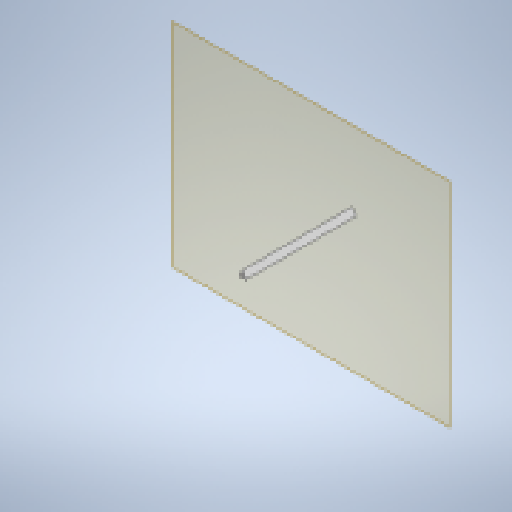
# Autodesk Inventor part: Pieza6
Saved by Autodesk Inventor 2024 (Build 280153000, 153)
## iProperties
Created: 2025-08-12
Part Number: Pieza6
Material: Genérico
Document SubType Name: Modeling
Designer: sergi
Density: 1 g/cm^3
Appearance: Valor por defecto
Author: sergi
Autodesk Inventor part; units mm, degrees
ref_plane "YZ Plane" through (0, 0, 0) normal (1, 0, 0) x (0, 1, 0)
ref_plane "XZ Plane" through (0, 0, 0) normal (0, 1, 0) x (-1, 0, 0)
ref_plane "XY Plane" through (0, 0, 0) normal (0, 0, 1) x (1, 0, 0)
ref_plane "Plano de trabajo1" through (-12.367, 0.0002, 0) normal (0, 0, 1) x (1, -0.0000342, 0)
sketch "Boceto1" plane through (-12.367, 0.0002, 0) normal (0, 0, 1) x (1, -0.0000342, 0)
  line L0 (0.0016, 0) -> (0.0463, 0.0894) projected
  line L1 (0.0016, 0) -> (0.1016, 0) projected
  line L2 (0.1016, 0) -> (0.0463, 0.0894)
  point P0 (12.367, 0.0002)
  constraints: 2 end point
extrude "Extrusión1" add sketch "Boceto1" along normal up to surface (1.5984 mm away)
